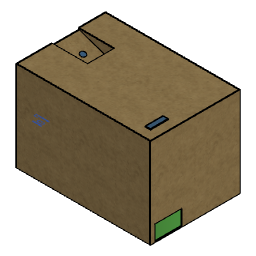
Lixeira Inteligente Sketchup (Autodesk Fusion 360 design; units mm, degrees)
Autodesk Fusion 360 part; units mm, degrees
sketch "Sketch4" plane through (0, 0, 0) normal (0, 0, 1) x (1, 0, 0)
  line L0 (0, 0) -> (750, 0)
  line L1 (750, 0) -> (750, 500)
  line L2 (750, 500) -> (0, 500)
  line L3 (0, 500) -> (0, 0)
  line L4 (5, 500) -> (5, 0)
  line L5 (745, 500) -> (745, 0)
  line L6 (5, 495) -> (745, 495)
  line L7 (5, 5) -> (745, 5)
  line L8 (5, 350) -> (745, 350)
  line L9 (5, 200) -> (745, 200)
  line L10 (5, 195) -> (745, 195)
  line L11 (5, 355) -> (745, 355)
  dimension "d16" = 750
  dimension "d17" = 500
  dimension "d18" = 5
  dimension "d19" = 5
  dimension "d20" = 5
  dimension "d21" = 5
  dimension "d23" = 150
  dimension "d24" = 200
  dimension "d25" = 250
  dimension "d26" = 5
  dimension "d27" = 5
  constraint horizontal L0
  constraint vertical L1
  constraint horizontal L2
  constraint vertical L3
  constraint coincident L0.start L3.end
  constraint coincident L2 L4.start
  constraint coincident L0 L4.end
  constraint perpendicular L0 L4
  constraint coincident L2 L5.start
  constraint coincident L0 L5.end
  constraint perpendicular L0 L5
  constraint coincident L4 L6.start
  constraint coincident L5 L6.end
  constraint perpendicular L5 L6
  constraint coincident L4 L7.start
  constraint coincident L5 L7.end
  constraint perpendicular L5 L7
  constraint coincident L4 L8.start
  constraint coincident L5 L8.end
  constraint perpendicular L5 L8
  constraint coincident L4 L9.start
  constraint coincident L5 L9.end
  constraint perpendicular L5 L9
  constraint coincident L4 L10.start
  constraint coincident L5 L10.end
  constraint perpendicular L1 L10
  constraint coincident L4 L11.start
  constraint coincident L5 L11.end
  constraint perpendicular L1 L11
  measures "d16" distance of L0.start L0.end
  measures "d17" distance of L0.start L2.end
  measures "d18" distance of L3 L4
  measures "d19" distance of L1 L5
  measures "d20" distance of L2 L6
  measures "d21" distance of L0 L7
  measures "d23" distance of L2 L8
  measures "d24" distance of L0 L9
  measures "d26" distance of L9 L10
  measures "d27" distance of L8 L11
extrude "Extrude4" add sketch "Sketch4" along normal blind 500 contours L0 L2 L3 L4 makes body 1
extrude "Extrude5" add sketch "Sketch4" along normal blind 500 separate body contours L2 L4 L5 L6 makes body 2
extrude "Extrude6" add sketch "Sketch4" along normal blind 500 separate body contours L4 L5 L8 L11 makes body 3
extrude "Extrude7" add sketch "Sketch4" along normal blind 500 separate body contours L4 L5 L9 L10 makes body 4
extrude "Extrude8" add sketch "Sketch4" along normal blind 500 separate body contours L0 L4 L5 L7 makes body 5
extrude "Extrude9" add sketch "Sketch4" along normal blind 500 separate body contours L0 L1 L2 L5 makes body 6
move_face "OffsetFaces1" offset -5 2 faces at (251.6667, 353.3333, 0) (251.6667, 198.3333, 0) on bodies 3 4
extrude "Extrude10" add sketch "Sketch4" along normal blind 5 separate body contours L4 L5 L7 L10 | L4 L5 L9 L10 | L4 L5 L6 L11 | L4 L5 L8 L9 | L4 L5 L8 L11 makes body 7
sketch "Sketch5" plane through (0, 0, 500) normal (0, 0, 1) x (-1, 0, 0)
  line L0 (0, -500) -> (0, 0)
  line L1 (0, 0) -> (-5, 0)
  line L2 (-5, 0) -> (-5, -500)
  line L3 (-5, -500) -> (0, -500)
  line L4 (-5, -350) -> (0, -350)
  line L5 (-5, -200) -> (0, -200)
  line L6 (-750, -500) -> (0, -500)
  line L7 (0, 0) -> (-750, 0)
  dimension "d43" = 150
  dimension "d44" = 200
  constraint coincident L2 L4.start
  constraint coincident L0 L4.end
  constraint perpendicular L0 L4
  constraint coincident L2 L5.start
  constraint coincident L0 L5.end
  constraint perpendicular L0 L5
  measures "d43" distance of L4 L6
  measures "d44" distance of L5 L7
extrude "Extrude11" cut sketch "Sketch5" against normal blind 10 contours L0 L2 L4 L5 bodies 1
copy_body "CopyPasteBodies1" bodies 7 makes body 8
move_body "Move1" bodies 8 to x (1, 0, 0) y (0, 1, 0) z (0, 0, 1) at (0, 0, 495)
extrude "Extrude12" cut 2 faces at (251.6667, 353.3333, 500) (251.6667, 198.3333, 500) along direction (0, 0, -1) blind 5 on bodies 3 4 bodies 3 4
sketch "Sketch6" plane through (0, 0, 500) normal (0, 0, 1) x (-1, 0, 0)
  line L0 (-5, -495) -> (-5, -5)
  line L1 (-5, -5) -> (-745, -5)
  line L2 (-745, -5) -> (-745, -495)
  line L3 (-745, -495) -> (-5, -495)
  line L4 (-5, -350) -> (-745, -350)
  line L5 (-5, -200) -> (-745, -200)
  line L6 (-750, -500) -> (0, -500)
  line L7 (0, 0) -> (-750, 0)
  line L8 (-150, -200) -> (-150, -350)
  line L9 (0, -500) -> (0, 0)
  line L10 (-665, -155) -> (-695, -155)
  line L11 (-695, -155) -> (-695, -55)
  line L12 (-695, -55) -> (-665, -55)
  line L13 (-665, -55) -> (-665, -155)
  dimension "d52" = 150
  dimension "d53" = 200
  dimension "d54" = 150
  dimension "d65" = 30
  dimension "d66" = 100
  dimension "d67" = 50
  dimension "d68" = 50
  constraint coincident L0 L4.start
  constraint coincident L2 L4.end
  constraint perpendicular L2 L4
  constraint coincident L0 L5.start
  constraint coincident L2 L5.end
  constraint perpendicular L2 L5
  constraint coincident L5 L8.start
  constraint coincident L4 L8.end
  constraint perpendicular L4 L8
  constraint horizontal L10
  constraint vertical L11
  constraint horizontal L12
  constraint vertical L13
  measures "d52" distance of L4 L6
  measures "d53" distance of L5 L7
  measures "d54" distance of L8 L9
  measures "d65" distance of L10.start L10.end
  measures "d66" distance of L10.start L12.end
  measures "d67" distance of L2 L11
  measures "d68" distance of L1 L12
extrude "Extrude13" cut sketch "Sketch6" against normal blind 5 contours L0 L4 L5 L8 bodies 8
sketch "Sketch7" plane through (0, 195, 0) normal (0, -1, 0) x (1, 0, 0)
  line L0 (745, 495) -> (5, 495)
  line L1 (5, 495) -> (5, 5)
  line L2 (5, 5) -> (745, 5)
  line L3 (745, 5) -> (745, 495)
  line L4 (5, 245) -> (745, 245)
  line L5 (5, 240) -> (745, 240)
  dimension "d57" = 5
  dimension "d58" = 250
  constraint coincident L1 L4.start
  constraint coincident L3 L4.end
  constraint perpendicular L3 L4
  constraint coincident L1 L5.start
  constraint coincident L3 L5.end
  constraint perpendicular L3 L5
  measures "d57" distance of L4 L5
  measures "d58" distance of L0 L4
extrude "Extrude14" add sketch "Sketch7" along normal blind 190 separate body contours L1 L3 L4 L5 makes body 9
sketch "Sketch8" plane through (0, 355, 0) normal (0, 1, 0) x (-1, 0, 0)
  line L0 (-5, 495) -> (-745, 495)
  line L1 (-745, 495) -> (-745, 5)
  line L2 (-745, 5) -> (-5, 5)
  line L3 (-5, 5) -> (-5, 495)
  line L4 (-745, 250) -> (-5, 250)
  line L5 (-745, 245) -> (-5, 245)
  line L6 (-745, 500) -> (-5, 500)
  dimension "d61" = 5
  dimension "d62" = 250
  constraint coincident L1 L4.start
  constraint coincident L3 L4.end
  constraint perpendicular L3 L4
  constraint coincident L1 L5.start
  constraint coincident L3 L5.end
  constraint perpendicular L3 L5
  measures "d61" distance of L4 L5
  measures "d62" distance of L4 L6
extrude "Extrude15" add sketch "Sketch8" along normal blind 140 separate body contours L1 L3 L4 L5 makes body 10
extrude "Extrude16" add sketch "Sketch6" along normal blind 5 separate body contours L10 L11 L12 L13 makes body 11
sketch "Sketch9" plane through (0, 0, 505) normal (0, 0, 1) x (-1, 0, 0)
  line L0 (-665, -55) -> (-695, -55)
  line L1 (-695, -55) -> (-695, -155)
  line L2 (-695, -155) -> (-665, -155)
  line L3 (-665, -155) -> (-665, -55)
  line L4 (-667, -155) -> (-667, -55)
  line L5 (-665, -55) -> (-665, -155)
  line L6 (-693, -155) -> (-693, -55)
  line L7 (-695, -155) -> (-695, -55)
  line L8 (-667, -57) -> (-693, -57)
  line L9 (-695, -55) -> (-665, -55)
  line L10 (-667, -153) -> (-693, -153)
  line L11 (-665, -155) -> (-695, -155)
  dimension "d71" = 2
  dimension "d72" = 2
  dimension "d73" = 2
  dimension "d74" = 2
  constraint coincident L2 L4.start
  constraint coincident L0 L4.end
  constraint perpendicular L0 L4
  constraint coincident L2 L6.start
  constraint coincident L0 L6.end
  constraint perpendicular L0 L6
  constraint coincident L4 L8.start
  constraint coincident L6 L8.end
  constraint perpendicular L6 L8
  constraint coincident L4 L10.start
  constraint coincident L6 L10.end
  constraint perpendicular L6 L10
  measures "d71" distance of L4 L5
  measures "d72" distance of L6 L7
  measures "d73" distance of L8 L9
  measures "d74" distance of L10 L11
extrude "Extrude17" cut sketch "Sketch9" against normal blind 1 contours L4 L6 L8 L10 bodies 11
extrude "Extrude18" cut sketch "Sketch6" against normal blind 5 contours L10 L11 L12 L13 bodies 8
sketch "Sketch10" plane through (0, 350, 0) normal (0, -1, 0) x (1, 0, 0)
  line L0 (745, 495) -> (5, 495)
  line L1 (5, 495) -> (5, 5)
  line L2 (5, 5) -> (745, 5)
  line L3 (745, 5) -> (745, 495)
  line L4 (5, 490) -> (745, 490)
  line L5 (5, 245) -> (745, 245)
  line L6 (545, 245) -> (545, 490)
  line L7 (745, 245) -> (5, 5)
  line L8 (745, 245) -> (746.5425, 240.2439)
  line L9 (746.5425, 240.2439) -> (21.2072, 5)
  line L10 (745, 305) -> (5, 305)
  line L11 (5, 490) -> (545, 305)
  line L12 (545, 305) -> (543.3795, 300.2699)
  line L13 (543.3795, 300.2699) -> (5, 484.7147)
  line L14 (224, 73) -> (205, 73)
  line L15 (205, 73) -> (205, 30)
  line L16 (205, 30) -> (224, 30)
  line L17 (224, 30) -> (224, 73)
  line L18 (393, 85) -> (374, 85)
  line L19 (374, 85) -> (374, 128)
  line L20 (374, 128) -> (393, 128)
  line L21 (393, 128) -> (393, 85)
  line L22 (543, 140) -> (562, 140)
  line L23 (562, 140) -> (562, 183)
  line L24 (562, 183) -> (543, 183)
  line L25 (543, 183) -> (543, 140)
  dimension "d79" = 5
  dimension "d80" = 245
  dimension "d81" = 200
  dimension "d84" = 5
  dimension "d85" = 60
  dimension "d86" = 5
  dimension "d171" = 43
  dimension "d172" = 19
  dimension "d173" = 200
  dimension "d174" = 19
  dimension "d175" = 43
  dimension "d176" = 150
  dimension "d177" = 19
  dimension "d178" = 43
  dimension "d179" = 150
  dimension "d180" = 25
  dimension "d181" = 80
  dimension "d182" = 135
  constraint coincident L1 L4.start
  constraint coincident L3 L4.end
  constraint perpendicular L3 L4
  constraint coincident L1 L5.start
  constraint coincident L3 L5.end
  constraint perpendicular L3 L5
  constraint coincident L5 L6.start
  constraint coincident L4 L6.end
  constraint perpendicular L4 L6
  constraint coincident L1.end L2.start
  constraint perpendicular L7 L8
  constraint coincident L2 L9.end
  constraint perpendicular L8 L9
  constraint coincident L3 L10.start
  constraint coincident L1 L10.end
  constraint perpendicular L1 L10
  constraint coincident L6 L11.end
  constraint coincident L10 L11.end
  constraint perpendicular L11 L12
  constraint coincident L1 L13.end
  constraint perpendicular L12 L13
  constraint horizontal L14
  constraint vertical L15
  constraint horizontal L16
  constraint vertical L17
  constraint horizontal L18
  constraint vertical L19
  constraint horizontal L20
  constraint vertical L21
  constraint horizontal L22
  constraint vertical L23
  constraint horizontal L24
  constraint vertical L25
  measures "d79" distance of L0 L4
  measures "d80" distance of L4 L5
  measures "d81" distance of L3 L6
  measures "d84" distance of L5.end L8.end
  measures "d85" distance of L5 L10
  measures "d86" distance of L11.end L12.end
  measures "d171" distance of L14.start L16.end
  measures "d172" distance of L14.start L14.end
  measures "d173" distance of L1 L15
  measures "d174" distance of L18.start L18.end
  measures "d175" distance of L18.start L20.end
  measures "d176" distance of L17 L19
  measures "d177" distance of L22.start L22.end
  measures "d178" distance of L22.start L24.end
  measures "d179" distance of L21 L25
  measures "d180" distance of L2 L16
  measures "d181" distance of L2 L18
  measures "d182" distance of L2 L22
extrude "Extrude19" add sketch "Sketch10" along normal blind 150 separate body contours L1 L10 L11 L13 | L10 L12 L13 makes body 12
extrude "Extrude20" add sketch "Sketch10" along normal blind 150 separate body contours L3 L7 L9 L23 L24 | L7 L9 L23 L24 L25 | L7 L9 L20 L21 L25 | L2 L7 L9 L15 | L7 L9 L19 L20 L21 | L7 L9 L14 L15 L17 | L7 L9 L14 L17 L19 makes body 13
sketch "Sketch11" plane through (150.7623, 0, 440.0629) normal (0.3241, 0, 0.946023) x (0, 1, 0)
  line L0 (350, -416.7318) -> (350, 154.0791)
  line L1 (350, 154.0791) -> (200, 154.0791)
  line L2 (200, 154.0791) -> (200, -416.7318)
  line L3 (200, -416.7318) -> (350, -416.7318)
  line L4 (200, 54.0791) -> (350, 54.0791)
  line L5 (200, -125.9209) -> (350, -125.9209)
  line L6 (200, -265.9209) -> (350, -265.9209)
  circle A0 centre (275, 54.0791) radius 15
  circle A1 centre (275, -125.9209) radius 7.5
  circle A2 centre (275, -265.9209) radius 5
  circle A3 centre (275, 54.0791) radius 15.5
  circle A4 centre (275, -125.9209) radius 8
  circle A5 centre (275, -265.9209) radius 5.5
  dimension "d91" = 100
  dimension "d92" = 180
  dimension "d93" = 140
  dimension "d94" = 30
  dimension "d95" = 15
  dimension "d96" = 10
  dimension "d103" = 31
  dimension "d104" = 16
  dimension "d105" = 11
  constraint coincident L2 L4.start
  constraint coincident L0 L4.end
  constraint perpendicular L0 L4
  constraint coincident L2 L5.start
  constraint coincident L0 L5.end
  constraint perpendicular L0 L5
  constraint coincident L2 L6.start
  constraint coincident L0 L6.end
  constraint perpendicular L0 L6
  constraint midpoint L4 A0.centre
  constraint midpoint L5 A1.centre
  constraint midpoint L6 A2.centre
  constraint concentric A0 A3
  constraint concentric A1 A4
  constraint concentric A2 A5
  measures "d91" distance of L1 L4
  measures "d92" distance of L4 L5
  measures "d93" distance of L5 L6
  measures "d94" diameter of A0
  measures "d95" diameter of A1
  measures "d96" diameter of A2
  measures "d103" diameter of A3
  measures "d104" diameter of A4
  measures "d105" diameter of A5
extrude "Extrude24" cut sketch "Sketch11" against normal blind 5 contours L4 A0 A3 | L4 A0 A3 | L4 A0 | L4 A0 bodies 12
extrude "Extrude25" cut sketch "Sketch11" against normal blind 5 contours L5 A1 A4 | L5 A1 A4 | L5 A1 | L5 A1 bodies 12
extrude "Extrude26" cut sketch "Sketch11" against normal blind 5 contours L6 A2 A5 | L6 A2 A5 | L6 A2 | L6 A2 bodies 12
extrude "Extrude27" add sketch "Sketch11" along normal blind 1 separate body contours L6 A2 | L6 A2 makes body 14
extrude "Extrude28" add sketch "Sketch11" against normal blind 6.5 contours L6 A2 | L6 A2 bodies 14
extrude "Extrude29" add sketch "Sketch11" along normal blind 1 separate body contours L5 A1 | L5 A1 makes body 15
extrude "Extrude30" add sketch "Sketch11" against normal blind 9 contours L5 A1 | L5 A1 bodies 15
extrude "Extrude31" add sketch "Sketch11" along normal blind 1 separate body contours L4 A0 | L4 A0 makes body 16
extrude "Extrude32" add sketch "Sketch11" against normal blind 14 contours L4 A0 | L4 A0 bodies 16
extrude "Extrude33" add 1 faces at (402.4185, 276.4927, 346.9765) along direction (-0.3241, 0, -0.946023) blind 100 on bodies 14 bodies 14
thread "Thread1" "ISO Metric profile 10.0 M10x1 6g" major diameter 9.884 minor diameter 8.744 pitch 1 angle 60 resizes the face on face at (374.8731, 276.3542, 288.5855) from (367.8128, 275, 253.1264) to (400.2229, 275, 347.7287) on bodies 14
extrude "Extrude34" add 1 faces at (266.617, 271.4153, 390.8585) along direction (-0.3241, 0, -0.946023) blind 130 on bodies 15 bodies 15
thread "Thread2" "ISO Metric profile 15.0 M15x1 6g" major diameter 14.884 minor diameter 13.7405 pitch 1 angle 60 resizes the face on face at (261.9158, 272.9687, 353.7103) from (224.8364, 275, 267.7547) to (266.9695, 275, 390.7377) on bodies 15
extrude "Extrude35" add 1 faces at (93.4339, 271.8826, 444.9044) along direction (-0.3241, 0, -0.946023) blind 170 on bodies 16 bodies 16
thread "Thread3" "ISO Metric profile 30.0 M30x1.5 6g" major diameter 29.85 minor diameter 28.132 pitch 1.5 angle 60 resizes the face on face at (60.6613, 289.9814, 341.6175) from (39.9678, 275, 283.5218) to (95.0649, 275, 444.3456) on bodies 16
extrude "Extrude36" cut 1 faces at (368.2722, 276.5741, 252.9691) along direction (0.3241, 0, 0.946023) blind 25 on bodies 14 bodies 14
sketch "Sketch12" plane through (0, 350, 0) normal (0, -1, 0) x (1, 0, 0)
  line L0 (745, 495) -> (5, 495)
  line L1 (5, 495) -> (5, 5)
  line L2 (5, 5) -> (745, 5)
  line L3 (745, 5) -> (745, 495)
  line L4 (510, 360) -> (550, 360)
  line L5 (550, 360) -> (550, 340)
  line L6 (550, 340) -> (510, 340)
  line L7 (510, 340) -> (510, 360)
  dimension "d138" = 40
  dimension "d139" = 20
  dimension "d140" = 195
  dimension "d141" = 135
  constraint horizontal L4
  constraint vertical L5
  constraint horizontal L6
  constraint vertical L7
  measures "d138" distance of L4.start L4.end
  measures "d139" distance of L4.start L6.end
  measures "d140" distance of L3 L5
  measures "d141" distance of L0 L4
extrude "Extrude37" add sketch "Sketch12" along normal blind 2 separate body contours L4 L5 L6 L7 makes body 17
extrude "Extrude38" cut sketch "Sketch12" against normal blind 5 contours L4 L5 L6 L7 bodies 3
extrude "Extrude39" cut 1 faces at (43.7864, 268.4938, 282.2136) along direction (0.3241, 0, 0.946023) blind 184 on bodies 16 bodies 16
extrude "Extrude40" add 1 faces at (103.8993, 269.0389, 456.1178) along direction (-0.3241, 0, -0.946023) blind 94 on bodies 16 bodies 16
extrude "Extrude41" cut 1 faces at (224.4712, 272.765, 267.8799) along direction (0.3241, 0, 0.946023) blind 139 on bodies 15 bodies 15
extrude "Extrude42" add 1 faces at (269.5211, 272.765, 399.377) along direction (-0.3241, 0, -0.946023) blind 74 on bodies 15 bodies 15
extrude "Extrude43" cut 1 faces at (375.456, 273.4259, 276.9344) along direction (0.3241, 0, 0.946023) blind 82 on bodies 14 bodies 14
extrude "Extrude44" add 1 faces at (402.9509, 276.5741, 354.1935) along direction (-0.3241, 0, -0.946023) blind 69 on bodies 14 bodies 14
sketch "Sketch13" plane through (0, 348, 0) normal (0, -1, 0) x (1, 0, 0)
  line L0 (510, 340) -> (550, 340)
  line L1 (550, 340) -> (550, 360)
  line L2 (550, 360) -> (510, 360)
  line L3 (510, 360) -> (510, 340)
  line L4 (530, 360) -> (530, 340)
  circle A0 centre (519.0552, 350) radius 5
  circle A1 centre (540.9448, 350) radius 5
  dimension "d158" = 10
  constraint midpoint L2 L4.start
  constraint midpoint L0 L4.end
  constraint symmetric L4 A0 A1
  measures "d158" diameter of A0
extrude "Extrude45" add sketch "Sketch13" along normal blind 5 contours A0 bodies 17
extrude "Extrude46" add sketch "Sketch13" along normal blind 5 contours A1 bodies 17
sketch "Sketch14" plane through (0, 0, 5) normal (0, 0, 1) x (-1, 0, 0)
  line L0 (-5, -495) -> (-5, -5)
  line L1 (-5, -5) -> (-745, -5)
  line L2 (-745, -5) -> (-745, -495)
  line L3 (-745, -495) -> (-5, -495)
  line L4 (-745, -25) -> (-635, -25)
  line L5 (-635, -25) -> (-635, -175)
  line L6 (-635, -175) -> (-745, -175)
  line L7 (-745, -175) -> (-745, -25)
  line L8 (-745, -195) -> (-5, -195)
  dimension "d163" = 110
  dimension "d164" = 150
  dimension "d165" = 20
  dimension "d166" = 20
  constraint horizontal L4
  constraint vertical L5
  constraint horizontal L6
  constraint vertical L7
  constraint collinear L2 L7
  measures "d163" distance of L4.start L4.end
  measures "d164" distance of L4.start L6.end
  measures "d165" distance of L1 L4
  measures "d166" distance of L6 L8
extrude "Extrude47" add sketch "Sketch14" along normal blind 85 separate body contours L2 L4 L5 L6 L7 makes body 18
extrude "Extrude48" cut 1 faces at (745, 75, 33.3333) along direction (1, 0, 0) blind 5 on bodies 18 bodies 6
extrude "Extrude49" add sketch "Sketch10" along normal blind 40 separate body contours L7 L9 L23 L24 L25 | L7 L24 L25 | L9 L22 L23 L25 makes body 19
extrude "Extrude50" add sketch "Sketch10" along normal blind 40 separate body contours L7 L9 L19 L20 L21 | L7 L19 L20 | L9 L18 L19 L21 makes body 20
extrude "Extrude51" add sketch "Sketch10" along normal blind 40 separate body contours L7 L14 L15 | L7 L9 L14 L15 L17 | L9 L15 L16 L17 makes body 21
move_body "Move2" bodies 19 20 21 to x (1, 0, 0) y (0, 1, 0) z (0, 0, 1) at (0, 46, 0)
sketch "Sketch16" plane through (0, 356, 0) normal (0, -1, 0) x (1, 0, 0)
  line L0 (543, 183) -> (543, 140)
  line L1 (543, 140) -> (562, 140)
  line L2 (562, 140) -> (562, 183)
  line L3 (562, 183) -> (543, 183)
  circle A0 centre (552.5, 173) radius 5
  dimension "d189" = 10
  dimension "d190" = 10
  measures "d189" diameter of A0
  measures "d190" distance of L3 A0.centre
extrude "Extrude52" add sketch "Sketch16" along normal blind 2 contours A0 bodies 19
sketch "Sketch17" plane through (0, 356, 0) normal (0, -1, 0) x (1, 0, 0)
  line L0 (393, 128) -> (374, 128)
  line L1 (374, 128) -> (374, 85)
  line L2 (374, 85) -> (393, 85)
  line L3 (393, 85) -> (393, 128)
  circle A0 centre (383.5, 118) radius 5
  dimension "d193" = 10
  dimension "d194" = 10
  measures "d193" diameter of A0
  measures "d194" distance of L0 A0.centre
extrude "Extrude53" add sketch "Sketch17" along normal blind 2 contours A0 bodies 20
sketch "Sketch18" plane through (0, 356, 0) normal (0, -1, 0) x (1, 0, 0)
  line L0 (224, 30) -> (224, 73)
  line L1 (224, 73) -> (205, 73)
  line L2 (205, 73) -> (205, 30)
  line L3 (205, 30) -> (224, 30)
  circle A0 centre (214.5, 63) radius 5
  dimension "d197" = 10
  dimension "d198" = 10
  measures "d197" diameter of A0
  measures "d198" distance of L1 A0.centre
extrude "Extrude54" add sketch "Sketch18" along normal blind 2 contours A0 bodies 21
extrude "Extrude55" cut sketch "Sketch16" along normal blind 10 contours A0 bodies 3
extrude "Extrude56" cut sketch "Sketch17" along normal blind 10 contours A0 bodies 3
extrude "Extrude57" cut sketch "Sketch18" along normal blind 10 contours A0 bodies 3
fillet "Fillet1" radius 2 12 edges at (543, 376, 140) (562, 376, 140) (562, 376, 183) (543, 376, 183) (393, 376, 85) (374, 376, 85) (393, 376, 128) (374, 376, 128) (205, 376, 30) (205, 376, 73) (224, 376, 73) (224, 376, 30) on bodies 19 20 21
sketch "Sketch19" plane through (0, 0, 245) normal (0, 0, 1) x (-1, 0, 0)
  line L0 (-745, -195) -> (-5, -195)
  line L1 (-5, -195) -> (-5, -5)
  line L2 (-5, -5) -> (-745, -5)
  line L3 (-745, -5) -> (-745, -195)
  line L4 (-55, -73) -> (-123, -73)
  line L5 (-123, -73) -> (-123, -20)
  line L6 (-123, -20) -> (-55, -20)
  line L7 (-55, -20) -> (-55, -73)
  line L8 (-55, -160) -> (-255, -160)
  line L9 (-255, -160) -> (-255, -110)
  line L10 (-255, -110) -> (-55, -110)
  line L11 (-55, -110) -> (-55, -160)
  dimension "d208" = 68
  dimension "d209" = 53
  dimension "d210" = 15
  dimension "d211" = 50
  dimension "d212" = 200
  dimension "d213" = 50
  dimension "d214" = 50
  dimension "d215" = 35
  constraint horizontal L4
  constraint vertical L5
  constraint horizontal L6
  constraint vertical L7
  constraint horizontal L8
  constraint vertical L9
  constraint horizontal L10
  constraint vertical L11
  measures "d208" distance of L4.start L4.end
  measures "d209" distance of L4.start L6.end
  measures "d210" distance of L2 L6
  measures "d211" distance of L1 L7
  measures "d212" distance of L8.start L8.end
  measures "d213" distance of L8.start L10.end
  measures "d214" distance of L1 L11
  measures "d215" distance of L0 L8
extrude "Extrude58" add sketch "Sketch19" along normal blind 10 separate body contours L8 L9 L10 L11 makes body 22
extrude "Extrude59" add sketch "Sketch19" along normal blind 1 separate body contours L4 L5 L6 L7 makes body 23
sketch "Sketch20" plane through (0, 0, 246) normal (0, 0, 1) x (-1, 0, 0)
  line L0 (-55, -20) -> (-123, -20)
  line L1 (-123, -20) -> (-123, -73)
  line L2 (-123, -73) -> (-55, -73)
  line L3 (-55, -73) -> (-55, -20)
  line L4 (-65, -55) -> (-46.8283, -55)
  line L5 (-46.8283, -55) -> (-46.8283, -68.0358)
  line L6 (-46.8283, -68.0358) -> (-65, -68.0358)
  line L7 (-65, -68.0358) -> (-65, -55)
  line L8 (-115, -35) -> (-82.9177, -35)
  line L9 (-82.9177, -35) -> (-82.9177, -46.5)
  line L10 (-82.9177, -46.5) -> (-115, -46.5)
  line L11 (-115, -46.5) -> (-115, -35)
  line L12 (-118.7418, -68.0358) -> (-70, -68.0358)
  line L13 (-70, -68.0358) -> (-70, -65)
  line L14 (-70, -65) -> (-118.7418, -65)
  line L15 (-118.7418, -65) -> (-118.7418, -68.0358)
  line L16 (-118.7418, -23.4548) -> (-69.1189, -23.4548)
  line L17 (-69.1189, -23.4548) -> (-69.1189, -26.4548)
  line L18 (-69.1189, -26.4548) -> (-118.7418, -26.4548)
  line L19 (-118.7418, -26.4548) -> (-118.7418, -23.4548)
  dimension "d220" = 3
  constraint horizontal L4
  constraint vertical L5
  constraint horizontal L6
  constraint vertical L7
  constraint horizontal L8
  constraint vertical L9
  constraint horizontal L10
  constraint vertical L11
  constraint horizontal L12
  constraint vertical L13
  constraint horizontal L14
  constraint vertical L15
  constraint horizontal L16
  constraint vertical L17
  constraint horizontal L18
  constraint vertical L19
  measures "d220" distance of L16.start L18.end
extrude "Extrude60" add sketch "Sketch20" along normal blind 3 contours L8 L9 L10 L11 bodies 23
extrude "Extrude61" add sketch "Sketch20" along normal blind 10 contours L3 L4 L5 L6 | L3 L4 L6 L7 bodies 23
extrude "Extrude62" add sketch "Sketch20" along normal blind 5 contours L12 L13 L14 L15 | L16 L17 L18 L19 bodies 23
extrude "Extrude63" cut 1 faces at (150, 250, 498.3333) along direction (1, 0, 0) blind 50 on bodies 8 bodies 8
named bodies: "Frente", "Lado Tras", "Interno tras", "Interno Frente", "Lado Frente", "Tras", "Chao", "Teto", "Prateleira Frente", "Prateleira Tras", "Display", "Rampa Cima", "Rampa Baixo", "Sensor menor", "Sensor medio", "Sensor maoir", "Sensor Ultra", "Fonte", "alto", "medio", "baixo", "Protoboard", "Ardulino"
